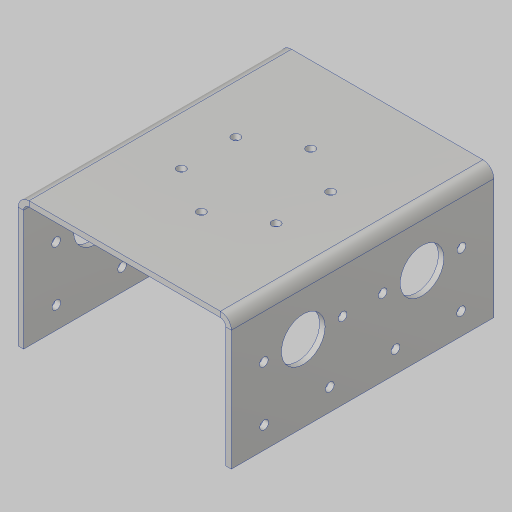
# Autodesk Inventor part: GP3-001
Saved by Autodesk Inventor 2023.5 (Build 275446000, 446)
## iProperties
Created: 2025-01-14
Part Number: GP3-001
Material: Aluminum 6061
Document SubType Name: Sheet Metal
Designer: brand
Density: 2.7 g/cm^3
Sheet Metal Rule: Default
Appearance: Aluminum - Flat
Mass: 327.405 g
Surface Area: 807.668 cm^2
Volume: 121.261 cm^3
Author: brand
Autodesk Inventor part; units mm, degrees
ref_plane "YZ Plane" through (0, 0, 0) normal (1, 0, 0) x (0, 1, 0)
ref_plane "XZ Plane" through (0, 0, 0) normal (0, 1, 0) x (-1, 0, 0)
ref_plane "XY Plane" through (0, 0, 0) normal (0, 0, 1) x (1, 0, 0)
sketch "Sketch1" plane through (0, 0, 0) normal (0, 1, 0) x (-1, 0, 0)
  line L0 (61.9125, -76.2) -> (-61.9125, -76.2)
  line L1 (-61.9125, -76.2) -> (-61.9125, 76.2)
  line L2 (-61.9125, 76.2) -> (61.9125, 76.2)
  line L3 (61.9125, 76.2) -> (61.9125, -76.2)
  line L4 (61.9125, -76.2) -> (-61.9125, 76.2) construction
  line L5 (-61.9125, -76.2) -> (61.9125, 76.2) construction
  point P0 (0, 0)
  dimension "d0" = 152.4
  dimension "d1" = 123.825
  measures "d0" distance of L2.end L0.start
  measures "d1" distance of L1.end L2.end
extrude "Plate1" add sketch "Sketch1" along normal mid plane 3.175
sketch "Sketch3" plane through (58.7375, 1.5875, 76.2) normal (1, 0, 0) x (0, 1, 0)
  line L0 (0, -152.4) -> (0, 0)
  line L1 (0, 0) -> (-76.2, 0)
  line L2 (-76.2, 0) -> (-76.2, -152.4)
  line L3 (-76.2, -152.4) -> (0, -152.4)
  constraints: 6 end point, 1 horizontal, 1 perpendicular, 1 vertical
edge flange "Flange1" height 76.2 angle 90 thickness 3.175 bend radius 3.175 thickness toward (1, 0, 0) relief straight relief width 3.175 relief depth 1.5875 corner gap 3.175 corner form 0 edges at (61.9125, -1.5875, 0) (-61.9125, -1.5875, 0) wall of the first edge with corners at (58.7375, 1.5875, -76.2) (58.7375, 1.5875, 76.2) (58.7375, -74.6125, 76.2) (58.7375, -74.6125, -76.2)
bend "Bend1"
corner "Corner1"
sketch "Sketch4" plane through (61.9125, -74.6125, 76.2) normal (1, 0, 0) x (0, 0, -1)
  line L0 (0, 76.2) -> (152.4, 76.2) construction
  line L1 (0, 0) -> (0, 69.85) construction
  line L2 (41.7068, 44.45) -> (110.6932, 44.45) construction
  point P0 (76.2, 74.6125)
  point P1 (76.2, 44.45)
  point P2 (76.2, 76.2)
  dimension "d14" = 31.75
  dimension "d15" = 68.9864
  constraints: 2 end point, 2 midpoint, 1 horizontal, 1 horizontal alignment, 1 vertical alignment
  measures "d14" distance from line of L2.start L0
  measures "d15" distance of L2.end L2.start
hole "Hole1" at (61.9125, -30.1625, 34.4932) at (61.9125, -30.1625, -34.4932) direction (-1, 0, 0) diameter 25.4 end through all
sketch "Sketch5" plane through (0, 1.5875, 0) normal (0, 1, 0) x (1, 0, 0)
  circle A0 centre (0, 0) radius 31.75 construction
  point P0 (0, 31.75)
  dimension "d24" = 63.5
  constraints: 2 vertical alignment, 1 coincident, 2 other
hole "Hole2" at (0, 1.5875, -31.75) direction (0, -1, 0) diameter 5.1054 end through all clearance for "Flat Head Machine Screw (82)" size "#10" standard "Ansi Unified Screw Threads"
pattern_circular "Circular Pattern1" count 6 over 360 about axis through (0, -10, 0) along (0, 1, 0) of "Hole2"
sketch "Sketch6" plane through (61.9125, -74.6125, 76.2) normal (1, 0, 0) x (0, 0, -1)
  line L0 (19.05, 12.7) -> (57.15, 12.7) construction
  line L1 (57.15, 12.7) -> (95.25, 12.7) construction
  line L2 (95.25, 12.7) -> (133.35, 12.7) construction
  line L3 (152.4, 0) -> (0, 0) projected
  point P0 (76.2, 74.6125)
  point P1 (76.2, 12.7)
  point P2 (76.2, 0)
  dimension "d35" = 38.1
  dimension "d36" = 38.1
  dimension "d37" = 38.1
  dimension "d38" = 12.7
  constraints: 6 end point, 3 horizontal alignment, 2 collinear, 2 midpoint, 1 horizontal, 1 vertical alignment
  measures "d35" distance of L0.start L0.end
  measures "d36" distance of L0.end L1.end
  measures "d37" distance of L1.end L2.end
  measures "d38" distance from line of L3 L0.end
hole "Hole3" at (61.9125, -61.9125, 57.15) at (61.9125, -61.9125, 19.05) at (61.9125, -61.9125, -19.05) at (61.9125, -61.9125, -57.15) direction (-1, 0, 0) diameter 5.1054 end through all clearance for "Flat Head Machine Screw (82)" size "#10" standard "Ansi Unified Screw Threads"
sketch "Sketch7" plane through (61.9125, -74.6125, 76.2) normal (1, 0, 0) x (0, 0, -1)
  circle A0 centre (95.25, 12.7) radius 2.5527 projected
  circle A1 centre (19.05, 12.7) radius 2.5527 projected
  circle A2 centre (57.15, 12.7) radius 2.5527 projected
  circle A3 centre (133.35, 12.7) radius 2.5527 projected
  circle A4 centre (41.7068, 44.45) radius 12.7 projected
  circle A5 centre (110.6932, 44.45) radius 12.7 projected
  line L0 (0, 69.85) -> (152.4, 69.85) projected
  line L1 (152.4, 69.85) -> (152.4, 0) projected
  line L2 (152.4, 0) -> (0, 0) projected
  line L3 (0, 0) -> (0, 69.85) projected
  line L4 (18.8468, 44.45) -> (64.5668, 44.45) construction
  line L5 (87.8332, 44.45) -> (133.5532, 44.45) construction
  point P0 (76.2, 74.6125)
  dimension "d46" = 45.72
  dimension "d47" = 45.72
  constraints: 5 horizontal alignment, 4 end point, 2 coincident, 2 horizontal, 2 midpoint
  measures "d46" distance of L4.start L4.end
  measures "d47" distance of L5.start L5.end
hole "Hole4" at (61.9125, -30.1625, 57.3532) at (61.9125, -30.1625, 11.6332) at (61.9125, -30.1625, -11.6332) at (61.9125, -30.1625, -57.3532) direction (-1, 0, 0) diameter 5.1054 end through all clearance for "Flat Head Machine Screw (82)" size "#10" standard "Ansi Unified Screw Threads"
equation "\"d22\" = Thickness"
equation "\"d30\" = Thickness"
equation "\"d36\" = d35"
equation "\"d37\" = d35"
equation "\"d44\" = Thickness"
equation "\"d47\" = d46"
equation "\"d53\" = Thickness"
equation "\"d2\" = Thickness"
equation "\"d4\" = BendReliefWidth"
equation "\"d5\" = BendReliefDepth"
equation "\"d6\" = MinimumRemnant"
equation "\"d7\" = TransitionRadius"
equation "\"d10\" = BendRadius"
equation "\"d11\" = CornerReliefSize"
equation "\"d12\" = GapSize"
equation "\"d13\" = JacobiRadiusSize"
equation "\"BendRadius\" = Thickness"
equation "\"BendReliefWidth\" = Thickness"
equation "\"BendReliefDepth\" = 0.5 * Thickness"
equation "\"CornerReliefSize\" = 4 * Thickness"
equation "\"MinimumRemnant\" = 2 * Thickness"
equation "\"TransitionRadius\" = BendRadius"
equation "\"JacobiRadiusSize\" = BendRadius"
equation "\"GapSize\" = Thickness"
equation "\"Thickness\" = 3.175"
body "Solid1"
